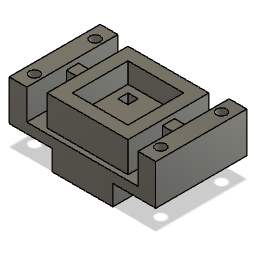
HW1 v1 (Autodesk Fusion 360 design; units mm, degrees)
Autodesk Fusion 360 part; units mm, degrees
sketch "Sketch1" plane through (0, 0, 0) normal (0, 1, 0) x (1, 0, 0)
  line L0 (72.5, -45) -> (-72.5, -45)
  line L1 (-72.5, -45) -> (-72.5, 45)
  line L2 (-72.5, 45) -> (72.5, 45)
  line L3 (72.5, 45) -> (72.5, -45)
  line L4 (72.5, -45) -> (-72.5, 45) construction
  line L5 (-72.5, -45) -> (72.5, 45) construction
  dimension "d1" = 145
  dimension "d2" = 90
  constraint horizontal L0
  constraint perpendicular L0 L1
  constraint parallel L0 L2
  constraint parallel L1 L3
  constraint coincident L4 origin
  constraint coincident L5 origin
  measures "d1" distance of L1.end L2.end
  measures "d2" distance of L0.end L1.end
extrude "Extrude1" add sketch "Sketch1" along normal blind 10
sketch "Sketch2" plane through (0, 10, 0) normal (0, 1, 0) x (-1, 0, 0)
  line L0 (-72.5, -45) -> (72.5, -45)
  line L1 (72.5, -45) -> (72.5, 45)
  line L2 (72.5, 45) -> (-72.5, 45)
  line L3 (-72.5, 45) -> (-72.5, -45)
  line L4 (72.5, -45) -> (55, -45)
  line L5 (55, -45) -> (55, 45)
  line L6 (55, 45) -> (72.5, 45)
  line L7 (72.5, 45) -> (72.5, -45)
  line L8 (-72.5, -45) -> (-55, -45)
  line L9 (-55, -45) -> (-55, 45)
  line L10 (-55, 45) -> (-72.5, 45)
  line L11 (-72.5, 45) -> (-72.5, -45)
  line L12 (-62.5, 30) -> (62.5, 30) construction
  line L13 (62.5, 30) -> (62.5, -30) construction
  line L14 (62.5, -30) -> (-62.5, -30) construction
  line L15 (-62.5, -30) -> (-62.5, 30) construction
  line L16 (-62.5, 30) -> (62.5, -30) construction
  line L17 (62.5, 30) -> (-62.5, -30) construction
  circle A0 centre (62.5, 30) radius 5
  circle A1 centre (-62.5, 30) radius 5
  circle A2 centre (62.5, -30) radius 5
  circle A3 centre (-62.5, -30) radius 5
  line L18 (-40, 40) -> (40, 40)
  line L19 (40, 40) -> (40, -40)
  line L20 (40, -40) -> (-40, -40)
  line L21 (-40, -40) -> (-40, 40)
  line L22 (-40, 40) -> (40, -40) construction
  line L23 (40, 40) -> (-40, -40) construction
  line L24 (-27.5, 27.5) -> (27.5, 27.5)
  line L25 (27.5, 27.5) -> (27.5, -27.5)
  line L26 (27.5, -27.5) -> (-27.5, -27.5)
  line L27 (-27.5, -27.5) -> (-27.5, 27.5)
  line L28 (-27.5, 27.5) -> (27.5, -27.5) construction
  line L29 (27.5, 27.5) -> (-27.5, -27.5) construction
  line L30 (-40, 6) -> (40, 6) construction
  line L31 (40, 6) -> (40, -6) construction
  line L32 (40, -6) -> (-40, -6) construction
  line L33 (-40, -6) -> (-40, 6) construction
  line L34 (-40, 6) -> (40, -6) construction
  line L35 (40, 6) -> (-40, -6) construction
  line L36 (-40, -6) -> (-55, -6)
  line L37 (-55, -6) -> (-55, 6)
  line L38 (-55, 6) -> (-40, 6)
  line L39 (-40, 6) -> (-40, -6)
  line L40 (40, -6) -> (55, -6)
  line L41 (55, -6) -> (55, 6)
  line L42 (55, 6) -> (40, 6)
  line L43 (40, 6) -> (40, -6)
  dimension "d5" = 17.5
  dimension "d6" = 90
  dimension "d7" = 17.5
  dimension "d8" = 90
  dimension "d9" = 125
  dimension "d10" = 60
  dimension "d11" = 10
  dimension "d14" = -125
  dimension "d15" = -60
  dimension "d16" = 80
  dimension "d17" = 80
  dimension "d18" = 55
  dimension "d19" = 55
  dimension "d20" = 80
  dimension "d21" = 12
  dimension "d22" = 12
  dimension "d23" = 12
  constraint horizontal L4
  constraint vertical L5
  constraint horizontal L6
  constraint vertical L7
  constraint coincident L0.end L1.start
  constraint horizontal L8
  constraint vertical L9
  constraint horizontal L10
  constraint vertical L11
  constraint coincident L0.start L3.end
  constraint horizontal L12
  constraint perpendicular L12 L13
  constraint parallel L12 L14
  constraint parallel L13 L15
  constraint coincident L16 origin
  constraint coincident L17 origin
  constraint coincident L12.end L13.start
  constraint horizontal L18
  constraint perpendicular L18 L19
  constraint parallel L18 L20
  constraint parallel L19 L21
  constraint coincident L22 origin
  constraint coincident L23 origin
  constraint horizontal L24
  constraint perpendicular L24 L25
  constraint parallel L24 L26
  constraint parallel L25 L27
  constraint coincident L28 origin
  constraint coincident L29 origin
  constraint horizontal L30
  constraint perpendicular L30 L31
  constraint parallel L30 L32
  constraint parallel L31 L33
  constraint coincident L34 origin
  constraint coincident L35 origin
  constraint horizontal L36
  constraint vertical L37
  constraint horizontal L38
  constraint vertical L39
  constraint coincident L9 L37.end
  constraint horizontal L40
  constraint vertical L41
  constraint horizontal L42
  constraint vertical L43
  measures "d5" distance of L0.end L4.end
  measures "d6" distance of L0.end L1.end
  measures "d7" distance of L0.start L8.end
  measures "d8" distance of L0.start L2.end
  measures "d9" distance of L13.end L14.end
  measures "d10" distance of L12.end L13.end
  measures "d11" diameter of A0
  measures "d16" distance of L19.end L20.end
  measures "d17" distance of L18.end L19.end
  measures "d18" distance of L25.end L26.end
  measures "d19" distance of L24.end L25.end
  measures "d20" distance of L31.end L32.end
  measures "d21" distance of L30.end L31.end
  measures "d22" distance of L32.end L30.start
  measures "d23" distance of L31.end L30.end
extrude "Extrude2" add sketch "Sketch2" along normal blind 30 contours L0 L2 L3 L8 L9 L10 L11 L37 | L0 L1 L2 L4 L5 L6 L7 L41 | L18 L19 L20 L21 L39 L43
extrude "Extrude3" cut sketch "Sketch2" against normal blind 10 contours A0 | A1 | A2 | A3
extrude "Extrude4" add sketch "Sketch2" along normal blind 10 contours L24 L25 L26 L27
extrude "Extrude5" add sketch "Sketch2" along normal blind 25 contours L9 L21 L36 L37 L38 L39 | L5 L19 L40 L41 L42 L43
sketch "Sketch3" plane through (0, 0, 0) normal (0, -1, 0) x (1, 0, 0)
  circle A0 centre (62.5, -30) radius 5
  circle A1 centre (-62.5, -30) radius 5
  circle A2 centre (62.5, 30) radius 5
  circle A3 centre (-62.5, 30) radius 5
  line L0 (-72.5, -45) -> (72.5, -45)
  line L1 (72.5, -45) -> (72.5, 45)
  line L2 (72.5, 45) -> (-72.5, 45)
  line L3 (-72.5, 45) -> (-72.5, -45)
  line L4 (30, 45) -> (-30, 45)
  line L5 (-30, 45) -> (-30, -45)
  line L6 (-30, -45) -> (30, -45)
  line L7 (30, -45) -> (30, 45)
  line L8 (30, 45) -> (-30, -45) construction
  line L9 (-30, 45) -> (30, -45) construction
  dimension "d32" = 60
  dimension "d33" = 90
  constraint horizontal L4
  constraint perpendicular L4 L5
  constraint parallel L4 L6
  constraint parallel L5 L7
  constraint coincident L8 origin
  constraint coincident L9 origin
  measures "d32" distance of L5.end L6.end
  measures "d33" distance of L4.end L5.end
extrude "Extrude6" add sketch "Sketch3" along normal blind 20 contours L0 L2 L4 L5 L6 L7
sketch "Sketch4" plane through (0, 20, 0) normal (0, 1, 0) x (-1, 0, 0)
  line L0 (-27.5, -27.5) -> (27.5, -27.5)
  line L1 (27.5, -27.5) -> (27.5, 27.5)
  line L2 (27.5, 27.5) -> (-27.5, 27.5)
  line L3 (-27.5, 27.5) -> (-27.5, -27.5)
  line L4 (-15, 15) -> (15, 15) construction
  line L5 (15, 15) -> (15, -15) construction
  line L6 (15, -15) -> (-15, -15) construction
  line L7 (-15, -15) -> (-15, 15) construction
  line L8 (-15, 15) -> (15, -15) construction
  line L9 (15, 15) -> (-15, -15) construction
  line L10 (10, -10) -> (20, -10)
  line L11 (20, -10) -> (20, -20)
  line L12 (20, -20) -> (10, -20)
  line L13 (10, -20) -> (10, -10)
  line L14 (10, -10) -> (20, -20) construction
  line L15 (20, -10) -> (10, -20) construction
  line L16 (-10, -20) -> (-20, -20)
  line L17 (-20, -20) -> (-20, -10)
  line L18 (-20, -10) -> (-10, -20) construction
  line L19 (-10, -10) -> (-10, -20)
  line L20 (-10, -10) -> (-20, -20) construction
  line L21 (-20, -10) -> (-10, -10)
  line L22 (20, 10) -> (10, 10)
  line L23 (10, 10) -> (10, 20)
  line L24 (10, 20) -> (20, 10) construction
  line L25 (20, 20) -> (20, 10)
  line L26 (20, 20) -> (10, 10) construction
  line L27 (10, 20) -> (20, 20)
  line L28 (-10, 10) -> (-20, 10)
  line L29 (-20, 10) -> (-20, 20)
  line L30 (-20, 20) -> (-10, 10) construction
  line L31 (-10, 20) -> (-10, 10)
  line L32 (-10, 20) -> (-20, 10) construction
  line L33 (-20, 20) -> (-10, 20)
  point P0 (15, -15)
  point P1 (-15, -15)
  point P2 (-15, -15)
  point P3 (15, 15)
  point P4 (15, 15)
  point P5 (-15, 15)
  point P6 (-15, 15)
  dimension "d36" = 30
  dimension "d37" = 30
  dimension "d38" = 10
  dimension "d39" = 10
  dimension "d42" = -30
  dimension "d43" = 30
  constraint horizontal L4
  constraint perpendicular L4 L5
  constraint parallel L4 L6
  constraint parallel L5 L7
  constraint coincident L8 origin
  constraint coincident L9 origin
  constraint horizontal L10
  constraint perpendicular L10 L11
  constraint parallel L10 L12
  constraint parallel L11 L13
  constraint coincident L14 P0
  constraint coincident L15 P0
  constraint coincident P0 L5.end
  measures "d36" distance of P0 P2
  measures "d37" distance of P4 P0
  measures "d38" distance of L11.end L12.end
  measures "d39" distance of L10.end L11.end
extrude "Extrude7" cut sketch "Sketch4" against normal blind 40 contours L10 L11 L12 L13 | L16 L17 L19 L21 | L22 L23 L25 L27 | L28 L29 L31 L33
